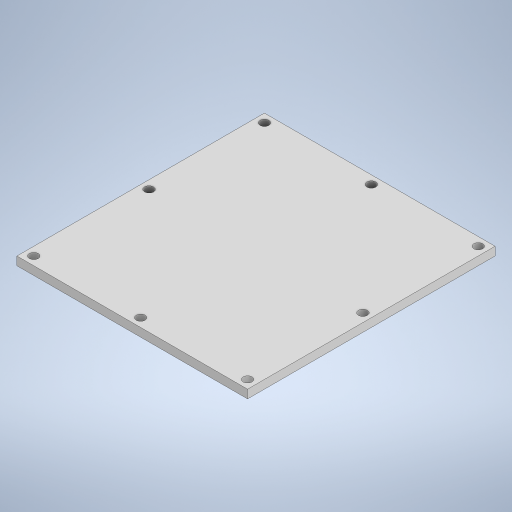
# Autodesk Inventor part: DummyBoard
Saved by Autodesk Inventor 2023 (Build 270158000, 158)
## iProperties
Created: 2022-08-17
Part Number: DummyBoard
Material: Generic
Document SubType Name: Modeling
Designer: Aditya Bansal
Density: 1 g/cm^3
Appearance: Default
Author: Aditya Bansal
Autodesk Inventor part; units mm, degrees
ref_plane "YZ Plane" through (0, 0, 0) normal (1, 0, 0) x (0, 1, 0)
ref_plane "XZ Plane" through (0, 0, 0) normal (0, 1, 0) x (-1, 0, 0)
ref_plane "XY Plane" through (0, 0, 0) normal (0, 0, 1) x (1, 0, 0)
sketch "Sketch1" plane through (0, 0, 0) normal (0, 1, 0) x (-1, 0, 0)
  line L0 (0, 0) -> (-82, 0)
  line L1 (-82, 0) -> (-82, -88)
  line L2 (-82, -88) -> (0, -88)
  line L3 (0, -88) -> (0, 0)
  dimension "d0" = 88
  dimension "d1" = 82
  constraints: 8 end point, 2 parallel, 1 horizontal, 1 perpendicular
  measures "d0" distance between parallel lines of L0 L2
  measures "d1" distance of L1.end L2.end
extrude "Extrusion1" add sketch "Sketch1" along normal blind 3
sketch "Sketch3" plane through (0, 3, 0) normal (0, 1, 0) x (1, 0, 0)
  line L0 (-0.75, 85.75) -> (82.75, 85.75) construction
  line L1 (82.75, 85.75) -> (82.75, 2.25) construction
  line L2 (82.75, 2.25) -> (-0.75, 2.25) construction
  line L3 (-0.75, 2.25) -> (-0.75, 85.75) construction
  line L4 (82, 0) -> (82, 88) projected
  line L5 (0, 88) -> (0, 0) projected
  line L6 (0, 0) -> (82, 0) projected
  line L7 (82, 88) -> (0, 88) projected
  point P0 (41, 85)
  point P1 (79, 44)
  point P2 (3, 44)
  point P3 (41, 3)
  point P4 (3, 85)
  point P5 (3, 3)
  point P6 (79, 3)
  point P7 (79, 85)
  dimension "d11" = 83.5
  dimension "d12" = 82
  dimension "d13" = 88
  dimension "d15" = 0.75
  dimension "d16" = 2.25
  dimension "d17" = 44
  dimension "d18" = 41
  dimension "d25" = 76
  dimension "d27" = 3
  dimension "d29" = 82
  dimension "d30" = 76
  dimension "d31" = 3
  dimension "d32" = 3
  dimension "d33" = 3
  dimension "d34" = 3
  constraints: 8 end point, 3 horizontal alignment, 3 vertical alignment, 2 parallel, 2 perpendicular, 1 horizontal
  measures "d11" distance of L0.end L1.end
  measures "d12" distance between parallel lines of L4 L5
  measures "d13" distance between parallel lines of L6 L7
  measures "d15" distance between parallel lines of L5 L3
  measures "d16" distance between parallel lines of L7 L0
  measures "d17" distance from line of L7 point (79, 44)
  measures "d18" distance from line of L4 point (41, 3)
  measures "d25" distance of point (79, 44) point (3, 44)
  measures "d27" distance from line of point (3, 44) L5
  measures "d29" distance of point (3, 85) point (3, 3)
  measures "d30" distance of point (79, 85) point (3, 85)
  measures "d31" distance from line of L7 point (3, 85)
  measures "d32" distance from line of point (3, 85) L5
  measures "d33" distance from line of L7 point (41, 85)
  measures "d34" distance from line of L6 point (41, 3)
hole "Hole1" at (41, 3, -85) at (79, 3, -44) at (3, 3, -44) at (41, 3, -3) at (3, 3, -85) at (79, 3, -85) at (3, 3, -3) at (79, 3, -3) direction (0, -1, 0) diameter 3.2 end through all clearance for "Flat Head Machine Screw" size "M3" standard "Ansi Metric M Profile"
equation "\"d15\" = -0.5 * d12 + 0.5 * d11"
equation "\"d16\" = -0.5 * d11 + 0.5 * d13"
equation "\"d17\" = 0.5 * d13"
equation "\"d18\" = 0.5 * d12"
equation "\"d27\" = -0.5 * d25 + 0.5 * d12"
equation "\"d31\" = -0.5 * d29 + 0.5 * d13"
equation "\"d32\" = -0.5 * d30 + 0.5 * d12"
equation "\"d34\" = d33"
body "Solid1"
